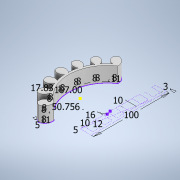
# Autodesk Inventor part: pneunet_approximate_test_first_bend_INFLATED
Saved by Autodesk Inventor 2021 (Build 250183000, 183)
## iProperties
Created: 2021-03-25
Part Number: pneunet_approximate_test_first_bend_INFLATED
Material: Generic
Document SubType Name: Modeling
Designer: Charlie
Density: 1 g/cm^3
Appearance: Default
Author: Charlie
Autodesk Inventor part; units mm, degrees
ref_plane "YZ Plane" through (0, 0, 0) normal (1, 0, 0) x (0, 1, 0)
ref_plane "XZ Plane" through (0, 0, 0) normal (0, 1, 0) x (-1, 0, 0)
ref_plane "XY Plane" through (0, 0, 0) normal (0, 0, 1) x (1, 0, 0)
sketch "Sketch1" plane through (0, 0, 0) normal (0, 1, 0) x (-1, 0, 0)
  line L0 (-34.333, 34.6818) -> (-49.333, 34.6818) construction
  line L1 (-34.333, -45.5191) -> (-34.333, 34.6818) construction
  line L2 (-34.333, 34.6818) -> (-49.333, -49.911) construction
  line L3 (-34.333, 34.6818) -> (-34.333, 29.6818) construction
  line L4 (-34.333, 19.6818) -> (-46.333, 19.6818) construction
  line L5 (-46.333, 19.6818) -> (-46.333, 29.6818) construction
  line L6 (-46.333, 29.6818) -> (-34.333, 29.6818) construction
  line L7 (-34.333, 3.6818) -> (-46.333, 3.6818) construction
  line L8 (-46.333, 3.6818) -> (-46.333, 13.6818) construction
  line L9 (-46.333, 13.6818) -> (-34.333, 13.6818) construction
  line L10 (-34.333, -12.3182) -> (-46.333, -12.3182) construction
  line L11 (-46.333, -12.3182) -> (-46.333, -2.3182) construction
  line L12 (-46.333, -2.3182) -> (-34.333, -2.3182) construction
  line L13 (-34.333, -28.3182) -> (-46.333, -28.3182) construction
  line L14 (-46.333, -28.3182) -> (-46.333, -18.3182) construction
  line L15 (-46.333, -18.3182) -> (-34.333, -18.3182) construction
  line L16 (-34.333, -44.3182) -> (-46.333, -44.3182) construction
  line L17 (-46.333, -44.3182) -> (-46.333, -34.3182) construction
  line L18 (-46.333, -34.3182) -> (-34.333, -34.3182) construction
  line L19 (-34.333, -60.3182) -> (-46.333, -60.3182) construction
  line L20 (-46.333, -60.3182) -> (-46.333, -50.3182) construction
  line L21 (-46.333, -50.3182) -> (-34.333, -50.3182) construction
  line L22 (-34.333, 19.6818) -> (-34.333, 13.6818) construction
  line L23 (-34.333, 3.6818) -> (-34.333, -2.3182) construction
  line L24 (-34.333, -12.3182) -> (-34.333, -18.3182) construction
  line L25 (-34.333, -28.3182) -> (-34.333, -34.3182) construction
  arc A0 (-7.5, -42.2964) -> (-7.5, 42.2964) centre (-35.5563, 0) ccw
  line L26 (-49.333, 34.6818) -> (-49.333, -65.3182) construction
  line L27 (-49.333, -65.3182) -> (-34.333, -65.3182) construction
  line L28 (-34.333, -65.3182) -> (-34.333, -60.3182) construction
  line L29 (0.7921, 54.796) -> (-7.5, 42.2964)
  line L30 (0.7921, 54.796) -> (4.9587, 52.032)
  line L31 (-1.8037, 41.8383) -> (4.9587, 52.032)
  line L32 (9.3874, 29.4913) -> (18.9468, 37.1243)
  line L33 (15.8269, 41.0315) -> (18.9468, 37.1243)
  line L34 (15.8269, 41.0315) -> (4.1052, 31.6719)
  line L35 (16.2597, 14.3103) -> (27.6972, 18.649)
  line L36 (25.9239, 23.3239) -> (27.6972, 18.649)
  line L37 (25.9239, 23.3239) -> (11.899, 18.0039)
  line L38 (18.1525, -2.2458) -> (30.3692, -1.6184)
  line L39 (30.1128, 3.375) -> (30.3692, -1.6184)
  line L40 (30.1128, 3.375) -> (15.1325, 2.6057)
  line L41 (14.8841, -18.5862) -> (26.706, -21.7303)
  line L42 (27.9911, -16.8982) -> (26.706, -21.7303)
  line L43 (27.9911, -16.8982) -> (13.495, -13.0429)
  line L44 (6.7685, -33.1405) -> (17.0595, -39.7539)
  line L45 (19.7626, -35.5476) -> (17.0595, -39.7539)
  line L46 (19.7626, -35.5476) -> (7.1437, -27.4381)
  line L47 (-5.4144, -44.51) -> (2.3568, -53.9573)
  line L48 (6.2182, -50.781) -> (2.3568, -53.9573)
  line L49 (6.2182, -50.781) -> (-3.3108, -39.1966)
  arc A1 (-5.4144, -44.51) -> (-5.8417, 44.7964) centre (-35.5563, 0) ccw
  line L50 (2.3568, -53.9573) -> (-7.329, -42.1825)
  arc A2 (0.7921, 54.796) -> (-7.5, 42.2964) centre (3.3515, 44.0979) ccw
  arc A3 (15.8269, 41.0315) -> (6.4495, 33.5438) centre (14.44, 33.1526) ccw
  arc A4 (9.3874, 29.4913) -> (18.9468, 37.1243) centre (10.9496, 37.3373) ccw
  arc A5 (25.9239, 23.3239) -> (14.704, 19.0679) centre (22.1907, 16.2484) ccw
  arc A6 (16.2597, 14.3103) -> (27.6972, 18.649) centre (20.1496, 21.301) ccw
  arc A7 (30.1128, 3.375) -> (18.1286, 2.7595) centre (24.3921, -2.2173) ccw
  arc A8 (18.1525, -2.2458) -> (30.3692, -1.6184) centre (23.9964, 3.2176) ccw
  arc A9 (27.9911, -16.8982) -> (16.3942, -13.814) centre (20.8326, -20.4699) ccw
  arc A10 (14.8841, -18.5862) -> (26.706, -21.7303) centre (22.1204, -15.1749) ccw
  arc A11 (19.7626, -35.5476) -> (9.6675, -29.06) centre (11.8543, -36.7553) ccw
  arc A12 (6.7685, -33.1405) -> (17.0595, -39.7539) centre (14.7018, -32.1092) ccw
  arc A13 (6.2182, -50.781) -> (-1.405, -41.5135) centre (-1.68, -49.5088) ccw
  arc A14 (-7.329, -42.1825) -> (2.3568, -53.9573) centre (3.6382, -43.0322) ccw
  arc A15 (-1.8037, 41.8383) -> (4.9587, 52.032) centre (-2.7195, 49.7857) ccw
  point P0 (0, 0)
  point P1 (-34.333, -5.4186)
  point P2 (-1.405, -41.5135)
  point P3 (9.6675, -29.06)
  point P4 (16.3942, -13.814)
  point P5 (18.1286, 2.7595)
  point P6 (14.704, 19.0679)
  point P7 (6.4495, 33.5438)
  point P8 (-7.5, 42.2964)
  dimension "d4" = 5
  dimension "d5" = 10
  dimension "d6" = 12
  dimension "d9" = 16
  dimension "d14" = 10
  dimension "d19" = 100
  dimension "d20" = 3
  dimension "d25" = 5
  dimension "d28" = 107
  dimension "d30" = 17.833
  dimension "d31" = 50.7557
  dimension "d32" = 11
  dimension "d34" = 8
  dimension "d35" = 8
  dimension "d36" = 8
  dimension "d37" = 8
  dimension "d38" = 8
  dimension "d39" = 8
  dimension "d40" = 8
  dimension "d41" = 8
  dimension "d42" = 8
  dimension "d43" = 8
  dimension "d44" = 8
  dimension "d46" = 11
  dimension "d47" = 8
  constraints: 102 end point, 31 point on circle, 15 centre point, 8 point on line, 4 equal length, 3 perpendicular, 2 vertical, 1 horizontal, 1 midpoint, 89 other
  measures "d4" distance of L0.start L3.end
  measures "d5" distance of L3.end L4.start
  measures "d6" distance of L4.start L4.end
  measures "d9" distance of L4.start L7.start
  measures "d14" distance of L13.end L14.end
  measures "d19" distance of L0.end L26.end
  measures "d20" distance between parallel lines of L26 L20
  measures "d25" distance of L29.start L30.end
  measures "d30" angle of L40 L35
  measures "d31" radius of A0
  measures "d32" radius of A2
  measures "d34" radius of A3
  measures "d35" radius of A4
  measures "d36" radius of A5
  measures "d37" radius of A6
  measures "d38" radius of A7
  measures "d39" radius of A8
  measures "d40" radius of A9
  measures "d41" radius of A10
  measures "d42" radius of A11
  measures "d43" radius of A12
  measures "d44" radius of A13
  measures "d46" radius of A14
  measures "d47" radius of A15
extrude "Extrusion1" add sketch "Sketch1" along normal blind 20
body "Solid1"
